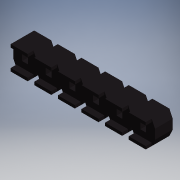
# Autodesk Inventor part: BF021-06-A-B-0400-0280-N-G_H
Saved by Autodesk Inventor 2017.3 (Build 213256000, 256)
## iProperties
Part Number: BF021-06-A-B-0400-0280-N-G_H
Material: Generic
Catalog Web Link: www.cadenas.de
Description: BF021 Housing-Header
Vendor: GCT
Document SubType Name: Modeling
Designer: partserver
Manufacturer: GCT
Mass: 0.0329084 g
Surface Area: 1.31405 cm^2
Volume: 0.0329084 cm^3
Density: 1 g/cm^3
Appearance: PSOLRGB-35-30-33
Category: PARTsolutions
Company: GCT
Title: BF021-06-A-B-0400-0280-N-G_H
Author: Cadenas PARTsolutions
Comments: Header
PSOL_IDENT_0: {$CADENAS_DATA\23d-libs\gct\b_t_b_connector\2_00mm\header\bf021\parts\bf021_header_housing.prj},228
PSOL_IDENT_1: {VTYP=3D},{NB=BF021-06-A-B-0400-0280-N-G_H},{LINA=BF021-06-A-B-0400-0280-N-G_H},{NN=BF021 Housing},{
PSOL_IDENT_2: DATE=06.12.2019 14:21:41},{GEOMDATE=22.02.2019 12:01:00},{VERSION=},{LINEID=10},{WBVAR=NOC,CP,W,C,D,
PSOL_IDENT_3: IM,PO},{WBNUMERIC=NOC,C,D}  {NB=BF021-06-A-B-0400-0280-N-G_H},{LINA=BF021-06-A-B-0400-0280-N-G_H},{K
PSOL_IDENT_4: T=DUMMY},{OC=BF021-06-A-B-0400-0280-N-G},{OCX=BF021},{NOC=6},{NOCX=6},{NOCXX=0},{CP=A},{W=B},{C=4.00
PSOL_IDENT_5: },{CX=4.00,[1.00:10.00]},{CCX1=400},{CEXX=0},{D=2.80},{DDX=2.80,[1:6]},{DEXX=0},{DEX1=280},{IM=N},{P
PSOL_IDENT_6: O=G},{POX= 'G', 'G = Plastic Box (Standard)','D', 'D = Tube', 'E'  , 'E = Tube with Cap'},{A=10.00},
PSOL_IDENT_7: {B=12.00},{OL=8.80},{WX=2.000},{DISCLAIMER=The creation and usage of 3D models generated by this bui
PSOL_IDENT_8: lder are covered in our disclaimer which can be viewed here}
NB: BF021-06-A-B-0400-0280-N-G_H
NN: BF021 Housing
NT: Header
NBSYN: $OC._H
LINA: BF021-06-A-B-0400-0280-N-G_H
CATALOG: Global Connector Technology
OC: BF021-06-A-B-0400-0280-N-G
NOC: 6
CP: A = Gold Flash All Over (Standard)
W: B = 2.00mm (Standard)
C: 4
D: 2.8
IM: N = Nylon 6T (Standard)
PO: G = Plastic Box (Standard)
A: 10
B: 12
DISCLAIMER: The creation and usage of 3D models generated by this builder are covered in our disclaimer which can be viewed here
SUPPLIER: GCT
ARTICLENO: BF021-06-A-B-0400-0280-N-G_H
BOMINFO: BF021-06-A-B-0400-0280-N-G_H
CREATOR: CADENAS GmbH
Autodesk Inventor part; units mm, degrees
sketch "Sketch_2" plane through (0, 0, 0) normal (0, 1, 0) x (-1, 0, 0)
  line L0 (1, -0.402) -> (1, 0.402)
  line L1 (1, 0.402) -> (0.7211, 1)
  line L2 (0.7211, 1) -> (-0.7211, 1)
  line L3 (-0.7211, 1) -> (-1, 0.402)
  line L4 (-1, 0.402) -> (-1, -0.402)
  line L5 (-1, -0.402) -> (-0.7211, -1)
  line L6 (-0.7211, -1) -> (0.7211, -1)
  line L7 (0.7211, -1) -> (1, -0.402)
  constraints: 16 end point
extrude "Extrusion1" add sketch "Sketch_2" along normal blind 2
pattern_linear "Rectangular Pattern1" count 6 spacing 2 along (1, 0, 0) of "Extrusion1"
sketch "Sketch_6" plane through (-1, 0, 0) normal (1, 0, 0) x (0, 0, -1)
  line L0 (-0.75, 0.5) -> (-0.75, 0)
  line L1 (-0.75, 0) -> (0.75, 0)
  line L2 (0.75, 0) -> (0.75, 0.5)
  line L3 (0.75, 0.5) -> (-0.75, 0.5)
  constraints: 8 end point
extrude "Extrusion2" cut sketch "Sketch_6" along normal blind 12
sketch "Sketch_4" plane through (0, 0, 0) normal (0, 1, 0) x (-1, 0, 0)
  line L0 (0.25, -0.25) -> (0.25, 0.25)
  line L1 (0.25, 0.25) -> (-0.25, 0.25)
  line L2 (-0.25, 0.25) -> (-0.25, -0.25)
  line L3 (-0.25, -0.25) -> (0.25, -0.25)
  constraints: 8 end point
extrude "Extrusion3" cut sketch "Sketch_4" along normal blind 2
pattern_linear "Rectangular Pattern2" count 6 spacing 2 along (1, 0, 0) of "Extrusion3"
sketch "Sketch_9" plane through (0, 0, 0) normal (0, 0, 1) x (1, 0, 0)
  line L0 (-1.28, 0.5) -> (-1.28, 0)
  line L1 (-1.28, 0) -> (-0.72, 0)
  line L2 (-0.72, 0) -> (-0.72, 0.5)
  line L3 (-0.72, 0.5) -> (-1.28, 0.5)
  constraints: 8 end point
extrude "Extrusion4" cut sketch "Sketch_9" along normal mid plane 2
pattern_linear "Rectangular Pattern3" count 7 spacing 2 along (1, 0, 0) of "Extrusion4"
ref_plane "FOR_PIN_1_XY" through (0, 2, 0) normal (0, 1, 0) x (1, 0, 0)
ref_plane "FOR_PIN_1_YZ" through (0, 2, 0) normal (1, 0, 0) x (0, 0, -1)
ref_plane "FOR_PIN_1_ZX" through (0, 2, 0) normal (0, 0, -1) x (0, 1, 0)
ref_plane "FOR_PIN_2_XY" through (2, 2, 0) normal (0, 1, 0) x (1, 0, 0)
ref_plane "FOR_PIN_2_YZ" through (2, 2, 0) normal (1, 0, 0) x (0, 0, -1)
ref_plane "FOR_PIN_2_ZX" through (2, 2, 0) normal (0, 0, -1) x (0, 1, 0)
ref_plane "FOR_PIN_3_XY" through (4, 2, 0) normal (0, 1, 0) x (1, 0, 0)
ref_plane "FOR_PIN_3_YZ" through (4, 2, 0) normal (1, 0, 0) x (0, 0, -1)
ref_plane "FOR_PIN_3_ZX" through (4, 2, 0) normal (0, 0, -1) x (0, 1, 0)
ref_plane "FOR_PIN_4_XY" through (6, 2, 0) normal (0, 1, 0) x (1, 0, 0)
ref_plane "FOR_PIN_4_YZ" through (6, 2, 0) normal (1, 0, 0) x (0, 0, -1)
ref_plane "FOR_PIN_4_ZX" through (6, 2, 0) normal (0, 0, -1) x (0, 1, 0)
ref_plane "FOR_PIN_5_XY" through (8, 2, 0) normal (0, 1, 0) x (1, 0, 0)
ref_plane "FOR_PIN_5_YZ" through (8, 2, 0) normal (1, 0, 0) x (0, 0, -1)
ref_plane "FOR_PIN_5_ZX" through (8, 2, 0) normal (0, 0, -1) x (0, 1, 0)
ref_plane "FOR_PIN_6_XY" through (10, 2, 0) normal (0, 1, 0) x (1, 0, 0)
ref_plane "FOR_PIN_6_YZ" through (10, 2, 0) normal (1, 0, 0) x (0, 0, -1)
ref_plane "FOR_PIN_6_ZX" through (10, 2, 0) normal (0, 0, -1) x (0, 1, 0)
ref_plane "IP_HOUSING_XY" through (-1, 0, 0) normal (0, 1, 0) x (1, 0, 0)
ref_plane "IP_HOUSING_YZ" through (-1, 0, 0) normal (1, 0, 0) x (0, 0, -1)
ref_plane "IP_HOUSING_ZX" through (-1, 0, 0) normal (0, 0, -1) x (0, 1, 0)
body "Solid1"
